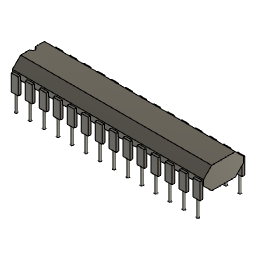
IC_DIP_28pin (Autodesk Fusion 360 design; units mm, degrees)
Autodesk Fusion 360 part; units mm, degrees
sketch "スケッチ1" plane through (0, 0, 0) normal (0, 0, 1) x (1, 0, 0)
  line L0 (-17.35, -3.65) -> (17.35, -3.65)
  line L1 (17.35, -3.65) -> (17.35, 3.65)
  line L2 (17.35, 3.65) -> (-17.35, 3.65)
  line L3 (-17.35, 3.65) -> (-17.35, -3.65)
  dimension "d1" = 34.7
  dimension "d2" = 7.3
  dimension "d23" = 17.35
  dimension "d24" = 3.65
  constraint horizontal L0
  constraint vertical L1
  constraint horizontal L2
  constraint vertical L3
  measures "d1" distance of L0.start L0.end
  measures "d2" distance of L0.start L2.end
  measures "d23" distance of origin L3
  measures "d24" distance of origin L0
extrude "押し出し1" add sketch "スケッチ1" along normal blind 4
chamfer "面取り1" distance 1.5 angle 45 4 edges at (0, -3.65, 4) (0, -3.65, 0) (0, 3.65, 4) (0, 3.65, 0)
sketch "スケッチ2" plane through (0, -3.65, 0) normal (0, -1, 0) x (1, 0, 0)
  line L0 (-17.35, 1.5) -> (17.35, 1.5)
  line L1 (17.35, 1.5) -> (17.35, 2.5)
  line L2 (17.35, 2.5) -> (-17.35, 2.5)
  line L3 (-17.35, 2.5) -> (-17.35, 1.5)
  line L4 (-17.15, 2.25) -> (-15.88, 2.25)
  line L5 (-15.88, 2.25) -> (-15.88, 1.75)
  line L6 (-15.88, 1.75) -> (-17.15, 1.75)
  line L7 (-17.15, 1.75) -> (-17.15, 2.25)
  dimension "d6" = 1.27
  dimension "d7" = 0.5
  dimension "d8" = 0.2
  dimension "d9" = 0.25
  constraint horizontal L4
  constraint vertical L5
  constraint horizontal L6
  constraint vertical L7
  measures "d6" distance of L4.start L4.end
  measures "d7" distance of L4.start L6.end
  measures "d8" distance of L3 L7
  measures "d9" distance of L0 L6
extrude "押し出し2" add sketch "スケッチ2" along normal blind 0.41 contours L4 L5 L6 L7
sketch "スケッチ3" plane through (0, 0, 1.75) normal (0, 0, -1) x (1, 0, 0)
  line L0 (-17.15, 3.65) -> (-15.88, 3.65)
  line L1 (-15.88, 3.65) -> (-15.88, 4.06)
  line L2 (-15.88, 4.06) -> (-17.15, 4.06)
  line L3 (-17.15, 4.06) -> (-17.15, 3.65)
  line L4 (-17.15, 4.06) -> (-15.88, 4.06)
  line L5 (-15.88, 4.06) -> (-15.88, 3.56)
  line L6 (-15.88, 3.56) -> (-17.15, 3.56)
  line L7 (-17.15, 3.56) -> (-17.15, 4.06)
  dimension "d12" = 0.5
  constraint horizontal L4
  constraint vertical L5
  constraint horizontal L6
  constraint vertical L7
  constraint coincident L2.end L3.start
  constraint coincident L1.end L5
  measures "d12" distance of L2.end L6.end
extrude "押し出し3" add sketch "スケッチ3" along normal blind 2.5
sketch "スケッチ4" plane through (0, 0, -0.75) normal (0, 0, -1) x (1, 0, 0)
  line L0 (-17.15, 3.56) -> (-15.88, 3.56)
  line L1 (-15.88, 3.56) -> (-15.88, 4.06)
  line L2 (-15.88, 4.06) -> (-17.15, 4.06)
  line L3 (-17.15, 4.06) -> (-17.15, 3.56)
  circle A0 centre (-16.515, 3.81) radius 0.25
  dimension "d15" = 0.5
  dimension "d16" = 0.635
  constraint tangent L2 A0
  measures "d15" diameter of A0
  measures "d16" distance of L3 A0.centre
extrude "押し出し4" add sketch "スケッチ4" along normal blind 3 contours A0
pattern_linear "R パターン1" count 14 spacing 2.54 along (1, 0, 0) of "押し出し2", "押し出し3", "押し出し4"
mirror "ミラー1" about plane through (0, 0, 0) normal (0, 1, 0) of "押し出し2", "押し出し3", "押し出し4", "R パターン1"
sketch "スケッチ5" plane through (0, 0, 4) normal (0, 0, 1) x (-1, 0, 0)
  line L0 (-17.35, -2.15) -> (17.35, -2.15)
  line L1 (17.35, -2.15) -> (17.35, 2.15)
  line L2 (17.35, 2.15) -> (-17.35, 2.15)
  line L3 (-17.35, 2.15) -> (-17.35, -2.15)
  arc A0 (17.35, 0.5) -> (17.35, -0.5) centre (17.35, 0) ccw
  line L4 (17.35, 0) -> (17.35, 0.5) construction
  line L5 (17.35, 0) -> (17.35, -0.5) construction
  dimension "d26" = 0.5
  dimension "d27" = 180
  constraint midpoint L1 A0.centre
  measures "d26" radius of A0
  measures "d27" angle of L4 L5
extrude "押し出し5" cut sketch "スケッチ5" against normal blind 0.5 contours L1 A0
